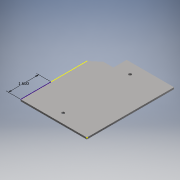
# Autodesk Inventor part: flywheel plate
Saved by Autodesk Inventor 2017 (Build 210142000, 142)
## iProperties
Created: 2016-10-19
Part Number: flywheel plate
Material: Steel, Alloy
Document SubType Name: Modeling
Designer: Aditya
Density: 7.73 g/cm^3
Appearance: Semi-Polished
Author: Aditya
Autodesk Inventor part; units mm, degrees
ref_plane "YZ Plane" through (0, 0, 0) normal (1, 0, 0) x (0, 1, 0)
ref_plane "XZ Plane" through (0, 0, 0) normal (0, 1, 0) x (-1, 0, 0)
ref_plane "XY Plane" through (0, 0, 0) normal (0, 0, 1) x (1, 0, 0)
sketch "Sketch1" plane through (0, 0, 0) normal (0, 1, 0) x (-1, 0, 0)
  line L0 (0, 0) -> (0, -116.84)
  line L1 (0, -116.84) -> (63.5, -116.84)
  line L2 (63.5, -116.84) -> (63.5, -99.06)
  line L3 (63.5, -99.06) -> (76.708, -99.06)
  line L4 (0, 0) -> (88.9, 0)
  line L5 (88.9, 0) -> (88.9, -88.9)
  line L6 (88.9, -88.9) -> (76.708, -99.06)
  circle A0 centre (44.45, -12.7) radius 1.905
  circle A1 centre (44.45, -102.235) radius 1.905
  dimension "d0" = 116.84
  dimension "d1" = 63.5
  dimension "d2" = 17.78
  dimension "d3" = 13.208
  dimension "d4" = 88.9
  dimension "d6" = 88.9
  constraints: 14 end point, 3 perpendicular, 2 centre point, 2 vertical, 1 horizontal
  measures "d0" distance of L0.start L0.end
  measures "d1" distance of L0.end L1.end
  measures "d2" distance of L1.end L2.end
  measures "d3" distance of L2.end L3.end
  measures "d4" distance of L0.start L4.end
  measures "d6" distance of L4.end L5.end
extrude "Extrusion1" add sketch "Sketch1" along normal blind 2.286
sketch "Sketch2" plane through (0, 2.286, 0) normal (0, 1, 0) x (1, 0, 0)
  line L0 (-88.9, 88.9) -> (-88.9, 0) projected
  line L1 (-88.9, 0) -> (-88.9, 40.64)
  point P0 (0, 0)
  dimension "d13" = 40.64
  constraints: 2 end point, 1 point on line
  measures "d13" distance of L0.end L1.end
sketch "Sketch3" plane through (0, 2.286, 0) normal (0, 1, 0) x (1, 0, 0)
  circle A0 centre (-85.09, 50.1764) radius 2.0193 projected
  circle A1 centre (-85.09, 69.2264) radius 2.0193 projected
  point P0 (0, 0)
extrude "Extrusion2" cut sketch "Sketch3" against normal blind 19.05
body "Solid1"
